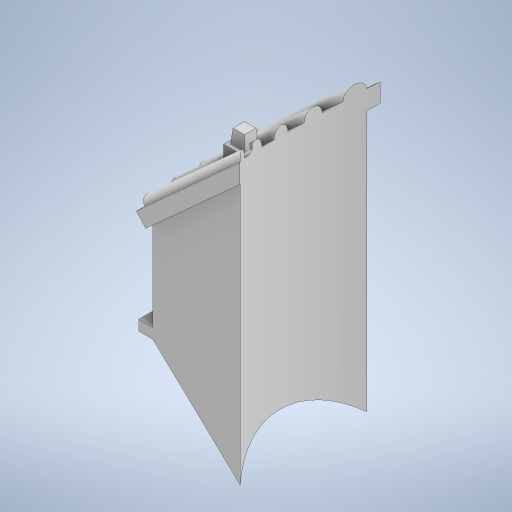
# Autodesk Inventor part: 另屋1 物1
Saved by Autodesk Inventor 2024 (Build 280153000, 153)
## iProperties
Created: 2024-05-24
Part Number: 另屋1 物1
Material: 一般
Document SubType Name: Modeling
Designer: User
Density: 1 g/cm^3
Appearance: 預設
Author: User
Autodesk Inventor part; units mm, degrees
ref_plane "YZ Plane" through (0, 0, 0) normal (1, 0, 0) x (0, 1, 0)
ref_plane "XZ Plane" through (0, 0, 0) normal (0, 1, 0) x (-1, 0, 0)
ref_plane "XY Plane" through (0, 0, 0) normal (0, 0, 1) x (1, 0, 0)
sketch "草圖1" plane through (0, 0, 0) normal (0, 0, 1) x (1, 0, 0)
  line L0 (0, 0) -> (13.5, 0)
  line L1 (0, 0) -> (0, 12.8)
  line L2 (0, 12.8) -> (13.5, 25.006146)
  line L3 (13.5, 0) -> (13.5, 25.006146)
  line L4 (0, 12.8) -> (-1.341335, 14.283516)
  line L5 (-1.341335, 14.283516) -> (13.5, 27.702442)
  line L6 (13.5, 27.702442) -> (13.5, 25.006146)
  dimension "d0" = 13.5
  dimension "d1" = 12.8
  dimension "d2" = 18.2
  dimension "d5" = 2
  constraints: 14 end point, 2 vertical, 1 collinear, 1 horizontal, 1 perpendicular
  measures "d0" distance of L0.start L0.end
  measures "d1" distance of L0.start L1.end
  measures "d2" distance of L2.end L1.end
  measures "d5" distance of L1.end L4.end
extrude "擠出1" add sketch "草圖1" along normal mid plane 18.2 contours L1 L2 L3 L0
extrude "擠出2" add sketch "草圖1" along normal mid plane 20.2 contours L4 L5 L6 L2
sketch "草圖2" plane through (0, 0, 9.1) normal (0, -1, 0) x (1, 0, 0)
  line L0 (10.315806, -5.875985) -> (7.315806, -5.875985)
  line L1 (7.315806, -5.875985) -> (7.315806, -2.875985)
  line L2 (7.315806, -2.875985) -> (10.315806, -2.875985)
  line L3 (10.315806, -2.875985) -> (10.315806, -5.875985)
  point P0 (0, -9.1)
  dimension "d8" = 3
  dimension "d9" = 3
  constraints: 8 end point, 2 parallel, 1 horizontal, 1 perpendicular
  measures "d8" distance of L1.end L2.end
  measures "d9" distance of L0.end L1.end
extrude "擠出3" add sketch "草圖2" against normal blind 25
sketch "草圖3" plane through (0, 25, 9.1) normal (0, 1, 0) x (1, 0, 0)
  line L0 (9.815806, 5.375985) -> (7.815806, 5.375985)
  line L1 (7.815806, 5.375985) -> (7.815806, 3.375985)
  line L2 (7.815806, 3.375985) -> (9.815806, 3.375985)
  line L3 (9.815806, 3.375985) -> (9.815806, 5.375985)
  line L4 (10.315806, 2.875985) -> (10.315806, 5.875985)
  line L5 (10.315806, 5.875985) -> (7.315806, 5.875985)
  point P0 (0, 9.1)
  dimension "d12" = 2
  dimension "d13" = 2
  dimension "d14" = 0.5
  dimension "d15" = 0.5
  constraints: 8 end point, 2 parallel, 1 horizontal, 1 perpendicular
  measures "d12" distance of L2.end L1.end
  measures "d13" distance of L1.end L0.end
  measures "d14" distance between parallel lines of L4 L3
  measures "d15" distance between parallel lines of L5 L0
extrude "擠出4" add sketch "草圖3" along normal blind 2 draft -5
sketch "草圖4" plane through (0, 0, -9.1) normal (-1, 0, 0) x (0, 0, 1)
  line L0 (0, 0) -> (18.2, 0)
  line L1 (18.2, 0) -> (18.2, -1.5)
  line L2 (18.2, -1.5) -> (0, -1.5)
  line L3 (0, -1.5) -> (0, 0)
  line L4 (18.2, 12.8) -> (18.2, 0) projected
  point P0 (9.1, 0)
  dimension "d18" = 18.2
  dimension "d19" = 1.5
  constraints: 8 end point, 2 parallel, 1 collinear, 1 horizontal, 1 perpendicular
  measures "d18" distance of L1.end L2.end
  measures "d19" distance of L0.end L1.end
extrude "擠出5" add sketch "草圖4" along normal blind 2 and the other way blind 13.5
sketch "草圖5" plane through (0, 12.8, -9.1) normal (-1, 0, 0) x (0, 0, 1)
  line L0 (18.2, -12.8) -> (0, -12.8)
  line L1 (4.086309, -12.8) -> (6.586309, -12.8)
  line L2 (5.336309, -12.8) -> (5.336309, -9.8)
  line L3 (4.336309, -12.8) -> (4.336309, -11.3)
  line L4 (6.336309, -12.8) -> (6.336309, -11.3)
  spline S0 degree 4 poles (4.086309, -12.8) (3.793492, -13.260986) (5.336309, -4.185352) (6.879126, -13.260986) (6.586309, -12.8) knots 0 0 0 0 0 1 1 1 1 1
  dimension "d24" = 2.5
  dimension "d25" = 3
  dimension "d26" = 1.5
  dimension "d27" = 1.5
  dimension "d28" = 1
  dimension "d29" = 1
  constraints: 8 end point, 4 point on line, 2 perpendicular, 1 midpoint, 1 vertical, 5 other
  measures "d24" distance of L1.start L1.end
  measures "d25" distance of L2.start L2.end
  measures "d26" distance of L3.start L3.end
  measures "d27" distance of L4.start L4.end
  measures "d28" distance between parallel lines of L2 L4
  measures "d29" distance between parallel lines of L2 L3
extrude "擠出6" add sketch "草圖5" along normal blind 0.5 contours L0 L4 S0 | L0 S0 | L0 L2 S0 L4 | L0 L3 S0 L2 | L0 S0 L3 picked at (6.603863, -12.809049)
sketch "草圖6" plane through (-0.5, 12.8, -9.1) normal (-1, 0, 0) x (0, 0, 1)
  line L0 (18.2, -12.8) -> (0, -12.8)
  line L1 (5.186405, -12.55) -> (5.186405, -12.05)
  line L2 (5.086405, -11.95) -> (4.586405, -11.95)
  line L3 (4.486405, -12.05) -> (4.486405, -12.55)
  line L4 (6.613905, -12.8) -> (4.058713, -12.8)
  line L5 (4.586405, -12.65) -> (5.086405, -12.65)
  line L6 (5.336405, -9.731293) -> (5.336405, -12.807466)
  line L7 (5.186405, -12.65) -> (4.486405, -12.65)
  line L8 (4.586405, -11.60072) -> (5.186405, -11.60072)
  line L9 (5.186405, -11.60072) -> (5.186405, -10.274322)
  spline S0 degree 4 poles (4.586405, -11.60072) (4.134277, -11.502296) (4.823095, -11.044584) (5.049571, -9.418647) (5.186405, -10.274322) knots 0 0 0 0 0 1 1 1 1 1
  arc A0 (4.586405, -11.95) -> (4.486405, -12.05) centre (4.586405, -12.05) ccw
  arc A1 (4.486405, -12.55) -> (4.586405, -12.65) centre (4.586405, -12.55) ccw
  arc A2 (5.086405, -12.65) -> (5.186405, -12.55) centre (5.086405, -12.55) ccw
  arc A3 (5.186405, -12.05) -> (5.086405, -11.95) centre (5.086405, -12.05) ccw
  line L10 (5.486405, -12.55) -> (5.486405, -12.05)
  line L11 (5.586405, -11.95) -> (6.086405, -11.95)
  line L12 (6.186405, -12.05) -> (6.186405, -12.55)
  line L13 (6.086405, -12.65) -> (5.586405, -12.65)
  line L14 (6.086405, -11.60072) -> (5.486405, -11.60072)
  line L15 (5.486405, -11.60072) -> (5.486405, -10.274322)
  spline S1 degree 4 poles (6.086405, -11.60072) (6.538533, -11.502296) (5.849715, -11.044584) (5.62324, -9.418647) (5.486405, -10.274322) knots 0 0 0 0 0 1 1 1 1 1
  arc A4 (6.186405, -12.05) -> (6.086405, -11.95) centre (6.086405, -12.05) ccw
  arc A5 (6.086405, -12.65) -> (6.186405, -12.55) centre (6.086405, -12.55) ccw
  arc A6 (5.486405, -12.55) -> (5.586405, -12.65) centre (5.586405, -12.55) ccw
  arc A7 (5.586405, -11.95) -> (5.486405, -12.05) centre (5.586405, -12.05) ccw
  point P0 (9.1, -12.8)
  point P1 (5.186405, -11.95)
  point P2 (4.486405, -11.95)
  point P3 (4.058713, -12.8)
  point P4 (4.447104, -11.467966)
  point P5 (4.686405, -10.804796)
  point P6 (5.059864, -10.063302)
  point P7 (5.486405, -11.95)
  point P8 (6.225707, -11.467966)
  point P9 (5.986405, -10.804796)
  point P10 (5.612947, -10.063302)
  dimension "d32" = 0.7
  dimension "d33" = 0.7
  dimension "d38" = 0.15
  dimension "d42" = 0.6
  dimension "d43" = 0.5
  dimension "d44" = 0.1
  dimension "d54" = 0.3
  dimension "d55" = 0.15
  dimension "d56" = 0.34928
  dimension "d57" = 1.7786
  dimension "d58" = 1.3
  dimension "d59" = 0.3
  dimension "d60" = 0.55308
  dimension "d61" = 0.4275
  dimension "d62" = 0.42769
  constraints: 28 end point, 19 symmetric about line, 16 point on circle, 11 point on line, 8 centre point, 8 tangent, 3 equal radius, 2 horizontal, 2 parallel, 1 perpendicular, 15 other
  measures "d32" distance of point (4.486, -11.95) point (5.186, -11.95)
  measures "d33" distance of L7.start point (5.186, -11.95)
  measures "d42" distance of L8.start L8.end
  measures "d43" distance from line of L9 point (4.686, -10.805)
  measures "d44" radius of A0
  measures "d54" distance between parallel lines of L15 L9
  measures "d55" distance between parallel lines of L6 L1
  measures "d56" distance between parallel lines of L2 L8
  measures "d57" distance of point (6.226, -11.468) point (4.447, -11.468)
  measures "d58" distance of point (5.986, -10.805) point (4.686, -10.805)
  measures "d59" distance of L15.end L9.end
  measures "d60" distance of point (5.613, -10.063) point (5.06, -10.063)
  measures "d61" distance from line of point (6.614, -12.8) L12
  measures "d62" distance from line of point (4.059, -12.8) L3
extrude "擠出7" cut sketch "草圖6" against normal blind 0.2
sketch "草圖7" plane through (0, 12.8, -9.1) normal (-1, 0, 0) x (0, 0, 1)
  line L0 (1.294579, -0.200276) -> (3.794579, -0.200276)
  line L1 (3.794579, -0.200276) -> (3.794579, -2.700276)
  line L2 (3.794579, -2.700276) -> (1.294579, -2.700276)
  line L3 (1.294579, -2.700276) -> (1.294579, -0.200276)
  line L4 (1.494579, -0.300276) -> (3.594579, -0.300276)
  line L5 (3.594579, -0.300276) -> (3.594579, -1.350276)
  line L6 (3.594579, -1.350276) -> (1.494579, -1.350276)
  line L7 (1.494579, -1.350276) -> (1.494579, -0.300276)
  line L8 (1.494579, -1.550276) -> (3.594579, -1.550276)
  line L9 (3.594579, -1.550276) -> (3.594579, -2.600276)
  line L10 (3.594579, -2.600276) -> (1.494579, -2.600276)
  line L11 (1.494579, -2.600276) -> (1.494579, -1.550276)
  point P0 (9.1, -12.8)
  dimension "d47" = 2.5
  dimension "d48" = 2.5
  dimension "d49" = 0.1
  dimension "d50" = 0.2
  dimension "d51" = 0.2
  dimension "d52" = 0.2
  dimension "d53" = 0.1
  constraints: 24 end point, 6 parallel, 3 horizontal, 3 perpendicular, 2 point on line, 1 collinear
  measures "d47" distance of L1.end L2.end
  measures "d48" distance of L0.end L1.end
  measures "d49" distance between parallel lines of L0 L4
  measures "d50" distance between parallel lines of L1 L5
  measures "d51" distance between parallel lines of L3 L7
  measures "d52" distance between parallel lines of L6 L8
  measures "d53" distance between parallel lines of L2 L10
extrude "擠出8" add sketch "草圖7" along normal blind 0.3
extrude "擠出9" cut sketch "草圖7" against normal blind 0.2 contours L4 L5 L6 L7 | L8 L9 L10 L11
sketch "草圖8" plane through (-1.341335, 14.283516, -10.1) normal (-0.7417582, -0.6706674, 0) x (0, 0, 1)
  line L0 (0, 0) -> (20.2, 0) projected
  line L1 (1, 0) -> (3, 0)
  line L2 (3, 0) -> (3, 1)
  line L3 (3, 1) -> (1, 1)
  line L4 (1, 1) -> (1, 0)
  line L5 (0, -2) -> (0, 0) projected
  line L6 (7, 0) -> (7, 1)
  line L7 (7, 1) -> (5, 1)
  line L8 (5, 1) -> (5, 0)
  line L9 (5, 0) -> (7, 0)
  line L10 (11, 0) -> (11, 1)
  line L11 (11, 1) -> (9, 1)
  line L12 (9, 1) -> (9, 0)
  line L13 (9, 0) -> (11, 0)
  line L14 (15, 0) -> (15, 1)
  line L15 (15, 1) -> (13, 1)
  line L16 (13, 1) -> (13, 0)
  line L17 (13, 0) -> (15, 0)
  line L18 (19, 0) -> (19, 1)
  line L19 (19, 1) -> (17, 1)
  line L20 (17, 1) -> (17, 0)
  line L21 (17, 0) -> (19, 0)
  point P0 (10.1, -11.494505)
  dimension "d67" = 2
  dimension "d68" = 1
  dimension "d69" = 1
  dimension "d72" = 4
  constraints: 40 end point, 2 horizontal, 2 parallel, 1 perpendicular, 1 point on line, 32 other
  measures "d67" distance of L3.end L2.end
  measures "d68" distance of L2.end L1.end
  measures "d69" distance between parallel lines of L5 L4
  measures "d72" distance of L1.end L6.start
extrude "擠出10" add sketch "草圖8" against normal up to surface surface through (13.5, 0, 0) normal (1, 0, 0)
fillet "圓角1" radius 1 10 edges at (5.744, 22.0379, -9.1) (5.744, 22.0379, -7.1) (5.744, 22.0379, -5.1) (5.744, 22.0379, -3.1) (5.744, 22.0379, -1.1) (5.744, 22.0379, 0.9) (5.744, 22.0379, 2.9) (2.6519, 19.2422, 4.9) (5.744, 22.0379, 6.9) (5.744, 22.0379, 8.9)
sketch "草圖9" plane through (0, 12.8, -9.1) normal (-1, 0, 0) x (0, 0, 1)
  line L0 (6, 1.483516) -> (8, 1.483516)
  line L1 (10, 1.483516) -> (12, 1.483516)
  line L2 (8, 2.415909) -> (10, 2.415909)
  line L3 (10, 2.415909) -> (10, -4.560157)
  line L4 (10, -4.560157) -> (8, -4.560157)
  line L5 (8, -4.560157) -> (8, 2.415909)
  line L6 (0, 0) -> (18.2, 0)
  arc A0 (10, 0.956327) -> (8, 0.956327) centre (9, 0.940622) ccw
  line L7 (8.2, -4.460157) -> (9.8, -4.460157)
  line L8 (9.8, -4.460157) -> (9.8, -3.289794)
  line L9 (9.8, -3.289794) -> (8.2, -3.289794)
  line L10 (8.2, -3.289794) -> (8.2, -4.460157)
  line L11 (8.2, -2.889794) -> (9.8, -2.889794)
  line L12 (9.8, -2.889794) -> (9.8, -0.984461)
  line L13 (9.8, -0.984461) -> (8.2, -0.984461)
  line L14 (8.2, -0.984461) -> (8.2, -2.889794)
  line L15 (8.2, -0.584461) -> (9.8, -0.584461)
  line L16 (9.8, -0.584461) -> (9.8, 0.940622)
  line L17 (8.2, 0.940622) -> (8.2, -0.584461)
  arc A1 (9.8, 0.940622) -> (8.2, 0.940622) centre (9, 0.940622) ccw
  point P0 (9.1, -12.8)
  point P1 (9.799846, 0)
  point P2 (8.200154, 0)
  point P3 (9.8, 0)
  point P4 (8.2, 0)
  point P5 (10, 0)
  point P6 (8, 0)
  dimension "d81" = 0.1
  dimension "d82" = 0.2
  dimension "d83" = 0.2
  dimension "d84" = 0.4
  dimension "d85" = 0.4
  dimension "d110" = 1.52508
  dimension "d111" = 1.90533
  dimension "d112" = 1.17036
  constraints: 30 end point, 6 perpendicular, 6 point on line, 5 parallel, 4 horizontal, 4 point on circle, 2 centre point, 2 tangent, 1 concentric
  measures "d81" distance between parallel lines of L4 L7
  measures "d82" distance between parallel lines of L3 L8
  measures "d83" distance between parallel lines of L5 L10
  measures "d84" distance between parallel lines of L9 L11
  measures "d85" distance between parallel lines of L13 L15
  measures "d110" distance from line of L15 A1.centre
  measures "d111" distance between parallel lines of L11 L13
  measures "d112" distance between parallel lines of L7 L9
extrude "擠出11" cut sketch "草圖9" along normal through all contours L6 L17 L15 L16 L3 L4 L5 | L17 A1 L16 L6 | L6 L16 L15 L17
extrude "擠出12" cut sketch "草圖9" against normal blind 0.2 contours L17 A1 L16 L6 | L6 L16 L15 L17 | L10 L9 L8 L7 | L14 L13 L12 L11
sketch "草圖11" plane through (0, 0, -9.1) normal (-1, 0, 0) x (0, 0, 1)
  line L0 (14.774456, 12.599724) -> (16.774456, 12.599724)
  line L1 (16.774456, 12.599724) -> (16.774456, 10.099724)
  line L2 (16.774456, 10.099724) -> (14.774456, 10.099724)
  line L3 (14.774456, 10.099724) -> (14.774456, 12.599724)
  line L4 (14.974456, 12.499724) -> (16.574456, 12.499724)
  line L5 (16.574456, 12.499724) -> (16.574456, 11.549724)
  line L6 (16.574456, 11.549724) -> (14.974456, 11.549724)
  line L7 (14.974456, 11.549724) -> (14.974456, 12.499724)
  line L8 (14.974456, 11.149724) -> (16.574456, 11.149724)
  line L9 (16.574456, 11.149724) -> (16.574456, 10.199724)
  line L10 (16.574456, 10.199724) -> (14.974456, 10.199724)
  line L11 (14.974456, 10.199724) -> (14.974456, 11.149724)
  line L12 (3.794579, 12.599724) -> (1.294579, 12.599724)
  point P0 (9.1, 0)
  dimension "d99" = 2
  dimension "d100" = 2.5
  dimension "d101" = 0.1
  dimension "d102" = 0.1
  dimension "d103" = 0.4
  dimension "d104" = 0.2
  dimension "d105" = 0.2
  constraints: 24 end point, 6 parallel, 3 horizontal, 3 perpendicular, 2 collinear, 2 point on line
  measures "d99" distance of L1.end L2.end
  measures "d100" distance of L0.end L1.end
  measures "d101" distance between parallel lines of L2 L10
  measures "d102" distance between parallel lines of L0 L4
  measures "d103" distance between parallel lines of L8 L6
  measures "d104" distance between parallel lines of L1 L5
  measures "d105" distance between parallel lines of L3 L7
extrude "擠出15" add sketch "草圖11" along normal blind 0.3
extrude "擠出16" cut sketch "草圖11" against normal blind 0.2 contours L4 L5 L6 L7 | L8 L9 L10 L11
extrude "擠出17" add sketch "草圖9" along normal blind 0.3 contours L6 L17 L15 L16 L3 L4 L5
sketch "草圖12" plane through (0, 0, 9.1) normal (0, 0, 1) x (1, 0, 0)
  line L0 (13.5, -1.5) -> (-2, -1.5)
  line L1 (0, -1.5) -> (13.5, -14.22717)
  line L2 (13.5, -14.22717) -> (13.5, -1.5)
  line L3 (13.5, -1.5) -> (0, -1.5)
  point P0 (0, 0)
  constraints: 6 end point, 1 collinear, 1 perpendicular, 1 point on line
extrude "擠出19" add sketch "草圖12" against normal up to surface (18.2 mm away)
sketch "草圖13" plane through (-2, 0, -9.1) normal (0, 1, 0) x (1, 0, 0)
  line L0 (15.5, 1) -> (2, 1)
  line L1 (15.5, -19.2) -> (15.5, -18.2)
  arc A0 (15.5, 1) -> (15.5, -19.2) centre (25.194844, -9.1) ccw
  line L2 (15.5, 1) -> (15.5, 0)
  line L3 (15.5, 1) -> (15.5, -19.2)
  point P0 (2, -9.1)
  dimension "d119" = 14
  constraints: 2 end point, 2 point on circle, 1 centre point, 1 vertical
  measures "d119" radius of A0
extrude "擠出20" cut sketch "草圖13" along normal through all both and the other way through all
